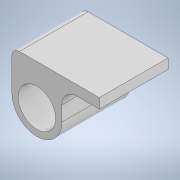
# Autodesk Inventor part: Деталь2
Saved by Autodesk Inventor 2021 (Build 250183000, 183)
## iProperties
Created: 2021-04-02
Part Number: Деталь2
Material: Типовые
Document SubType Name: Modeling
Designer: Данил
Density: 1 g/cm^3
Appearance: По умолчанию
Author: Данил
Autodesk Inventor part; units mm, degrees
ref_plane "YZ Plane" through (0, 0, 0) normal (1, 0, 0) x (0, 1, 0)
ref_plane "XZ Plane" through (0, 0, 0) normal (0, 1, 0) x (-1, 0, 0)
ref_plane "XY Plane" through (0, 0, 0) normal (0, 0, 1) x (1, 0, 0)
sketch "Эскиз3" plane through (0, 0, 0) normal (0, 0, 1) x (1, 0, 0)
  circle A0 centre (0, 0) radius 7.5
  circle A1 centre (0, 0) radius 10
  line L0 (-10, 0) -> (-10, 13)
  line L1 (-7, 16) -> (25, 16)
  line L2 (25, 16) -> (25, 12)
  line L3 (25, 12) -> (16, 12)
  arc A2 (-7, 16) -> (-10, 13) centre (-7, 13) ccw
  line L4 (10, 0) -> (10, 6)
  arc A3 (16, 12) -> (10, 6) centre (16, 6) ccw
  dimension "d15" = 15
  dimension "d16" = 20
  dimension "d17" = 3
  dimension "d18" = 4
  dimension "d19" = 6
  dimension "d20" = 35
  dimension "d21" = 16
  constraints: 10 end point, 6 point on circle, 4 centre point, 4 tangent, 3 vertical, 2 coincident, 2 horizontal alignment, 1 horizontal, 1 parallel
  measures "d15" diameter of A0
  measures "d16" diameter of A1
  measures "d17" radius of A2
  measures "d18" distance of L1.end L2.end
  measures "d19" radius of A3
  measures "d20" distance between parallel lines of L0 L2
  measures "d21" distance from line of L1 point (0, 0)
extrude "Выдавливание2" add sketch "Эскиз3" along normal mid plane 27.5
